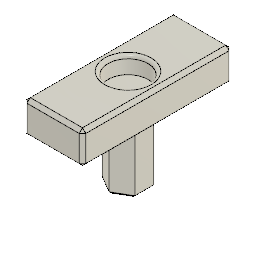
Hex Tool w magnet (Autodesk Fusion 360 design; units mm, degrees)
Autodesk Fusion 360 part; units mm, degrees
sketch "Sketch1" plane through (0, 0, 0) normal (0, 0, 1) x (1, 0, 0)
  line L0 (-2.5, -1.4434) -> (0, -2.8868)
  line L1 (0, -2.8868) -> (2.5, -1.4434)
  line L2 (2.5, -1.4434) -> (2.5, 1.4434)
  line L3 (2.5, 1.4434) -> (0, 2.8868)
  line L4 (0, 2.8868) -> (-2.5, 1.4434)
  line L5 (-2.5, 1.4434) -> (-2.5, -1.4434)
  dimension "d1" = 2.5
  constraint vertical L2
  measures "d1" distance of origin L5
extrude "Extrude1" add sketch "Sketch1" along normal blind 10 makes body 1
sketch "Sketch2" plane through (0, 0, 10) normal (0, 0, 1) x (-1, 0, 0)
  line L0 (2.5, -1.4434) -> (2.5, 1.4434)
  line L1 (2.5, 1.4434) -> (0, 2.8868)
  line L2 (0, 2.8868) -> (-2.5, 1.4434)
  line L3 (-2.5, 1.4434) -> (-2.5, -1.4434)
  line L4 (-2.5, -1.4434) -> (0, -2.8868)
  line L5 (0, -2.8868) -> (2.5, -1.4434)
  line L6 (2.5, -1.4434) -> (2.5, -11.4434)
  line L7 (2.5, -11.4434) -> (-2.5, -11.4434)
  line L8 (-2.5, -11.4434) -> (-2.5, -1.4434)
  line L9 (-2.5, 1.4434) -> (-2.5, 11.4434)
  line L10 (-2.5, 11.4434) -> (2.5, 11.4434)
  line L11 (2.5, 11.4434) -> (2.5, 1.4434)
  dimension "d4" = 5
  dimension "d5" = 5
  dimension "d6" = 10
  dimension "d7" = 10
  constraint coincident L0.start L5.end
  constraint vertical L6
  constraint perpendicular L6 L7
  constraint coincident L3.end L4.start
  constraint coincident L2.end L3.start
  constraint parallel L3 L9
  constraint perpendicular L9 L10
  constraint coincident L0.end L1.start
  measures "d4" distance of L9.end L10.end
  measures "d5" distance of L6.end L7.end
  measures "d6" distance of L10.end L0.end
  measures "d7" distance of L0.start L6.end
extrude "Extrude2" add sketch "Sketch2" along normal blind 5 separate body makes body 2
move_face "OffsetFaces1" offset 2 6 faces at (2.5, -0.4811, 11.6667) (2.5, 8.11, 11.6667) (2.5, -4.7767, 11.6667) (-2.5, 4.7767, 11.6667) (-2.5, 0.4811, 11.6667) (-2.5, -8.11, 11.6667) on bodies 2
combine "Combine1" operation add target body 1 tool bodies 2
sketch "Sketch3" plane through (0, 0, 15) normal (0, 0, 1) x (-1, 0, 0)
  line L0 (-4.5, 11.4434) -> (-4.5, -11.4434)
  line L1 (-4.5, -11.4434) -> (4.5, -11.4434)
  line L2 (4.5, -11.4434) -> (4.5, 11.4434)
  line L3 (4.5, 11.4434) -> (-4.5, 11.4434)
  circle A0 centre (0, 0) radius 3.05
  dimension "d11" = 6.1
  constraint coincident A0.centre origin
  measures "d11" diameter of A0
extrude "Extrude3" cut sketch "Sketch3" against normal blind 2.6 contours A0 bodies 1
fillet "Fillet1" radius 0.5 1 edges at (2.8436, -1.1029, 15) on bodies 1
chamfer "Chamfer1" distance 0.5 angle 45 12 edges at (0, -11.4434, 15) (4.5, 0, 15) (0, 11.4434, 15) (-4.5, 0, 15) (-4.5, 0, 10) (0, 11.4434, 10) (4.5, 0, 10) (4.5, -11.4434, 12.5) (0, -11.4434, 10) (4.5, 11.4434, 12.5) (-4.5, 11.4434, 12.5) (-4.5, -11.4434, 12.5) on bodies 1
chamfer "Chamfer2" distance 1 angle 45 6 edges at (1.25, -2.1651, 10) (2.5, 0, 10) (1.25, 2.1651, 10) (-1.25, 2.1651, 10) (-2.5, 0, 10) (-1.25, -2.1651, 10) on bodies 1
sketch "Sketch4" plane through (-4.5, 0, 0) normal (-1, 0, 0) x (0, -1, 0)
  line L0 (-10.9434, 10.5) -> (10.9434, 10.5)
  line L1 (10.9434, 10.5) -> (10.9434, 14.5)
  line L2 (10.9434, 14.5) -> (-10.9434, 14.5)
  line L3 (-10.9434, 14.5) -> (-10.9434, 10.5)
  spline S0 degree 2 poles (6.6137, 13.7758) (6.8028, 13.7758) (6.9498, 13.7019) knots 0 0 0 1 1 1
  spline S1 degree 2 poles (6.9498, 13.7019) (7.0968, 13.6279) (7.1888, 13.4869) knots 0 0 0 1 1 1
  spline S2 degree 2 poles (7.1888, 13.4869) (7.2808, 13.3459) (7.3117, 13.1482) knots 0 0 0 1 1 1
  line L4 (7.3117, 13.1482) -> (7.3117, 13.1465)
  line L5 (7.3117, 13.1465) -> (6.961, 13.1465)
  line L6 (6.961, 13.1465) -> (6.961, 13.1482)
  spline S3 degree 2 poles (6.961, 13.1482) (6.9421, 13.2858) (6.8509, 13.3623) knots 0 0 0 1 1 1
  spline S4 degree 2 poles (6.8509, 13.3623) (6.7598, 13.4388) (6.6137, 13.4388) knots 0 0 0 1 1 1
  spline S5 degree 2 poles (6.6137, 13.4388) (6.4452, 13.4388) (6.3532, 13.3262) knots 0 0 0 1 1 1
  spline S6 degree 2 poles (6.3532, 13.3262) (6.2612, 13.2135) (6.2612, 13.0089) knots 0 0 0 1 1 1
  line L7 (6.2612, 13.0089) -> (6.2612, 12.7992)
  spline S7 degree 2 poles (6.2612, 12.7992) (6.2612, 12.5963) (6.3532, 12.4837) knots 0 0 0 1 1 1
  spline S8 degree 2 poles (6.3532, 12.4837) (6.4452, 12.371) (6.6137, 12.371) knots 0 0 0 1 1 1
  spline S9 degree 2 poles (6.6137, 12.371) (6.7048, 12.371) (6.789, 12.4226) knots 0 0 0 1 1 1
  spline S10 degree 2 poles (6.789, 12.4226) (6.8733, 12.4742) (6.9369, 12.5671) knots 0 0 0 1 1 1
  line L8 (6.9369, 12.5671) -> (7.2567, 12.5671)
  line L9 (7.2567, 12.5671) -> (7.2567, 11.25)
  line L10 (7.2567, 11.25) -> (5.9826, 11.25)
  line L11 (5.9826, 11.25) -> (5.9826, 11.5836)
  line L12 (5.9826, 11.5836) -> (6.9059, 11.5836)
  line L13 (6.9059, 11.5836) -> (6.9059, 12.1458)
  spline S11 degree 2 poles (6.9059, 12.1458) (6.8406, 12.0925) (6.7598, 12.0633) knots 0 0 0 1 1 1
  spline S12 degree 2 poles (6.7598, 12.0633) (6.679, 12.034) (6.5947, 12.034) knots 0 0 0 1 1 1
  spline S13 degree 2 poles (6.5947, 12.034) (6.3781, 12.034) (6.2242, 12.1235) knots 0 0 0 1 1 1
  spline S14 degree 2 poles (6.2242, 12.1235) (6.0703, 12.2129) (5.9904, 12.3848) knots 0 0 0 1 1 1
  spline S15 degree 2 poles (5.9904, 12.3848) (5.9104, 12.5567) (5.9104, 12.7992) knots 0 0 0 1 1 1
  line L14 (5.9104, 12.7992) -> (5.9104, 13.0089)
  spline S16 degree 2 poles (5.9104, 13.0089) (5.9104, 13.2514) (5.9929, 13.4233) knots 0 0 0 1 1 1
  spline S17 degree 2 poles (5.9929, 13.4233) (6.0755, 13.5953) (6.2337, 13.6855) knots 0 0 0 1 1 1
  spline S18 degree 2 poles (6.2337, 13.6855) (6.3918, 13.7758) (6.6137, 13.7758) knots 0 0 0 1 1 1
  spline S19 degree 2 poles (3.2454, 12.6685) (3.2454, 12.4794) (3.3434, 12.3762) knots 0 0 0 1 1 1
  spline S20 degree 2 poles (3.3434, 12.3762) (3.4414, 12.273) (3.6185, 12.273) knots 0 0 0 1 1 1
  spline S21 degree 2 poles (3.6185, 12.273) (3.7818, 12.273) (3.8712, 12.3728) knots 0 0 0 1 1 1
  spline S22 degree 2 poles (3.8712, 12.3728) (3.9606, 12.4725) (3.9606, 12.6547) knots 0 0 0 1 1 1
  line L15 (3.9606, 12.6547) -> (4.0311, 12.3109)
  spline S23 degree 2 poles (4.0311, 12.3109) (3.9469, 12.1338) (3.8085, 12.0366) knots 0 0 0 1 1 1
  spline S24 degree 2 poles (3.8085, 12.0366) (3.67, 11.9395) (3.5033, 11.9395) knots 0 0 0 1 1 1
  spline S25 degree 2 poles (3.5033, 11.9395) (3.3107, 11.9395) (3.174, 12.0246) knots 0 0 0 1 1 1
  spline S26 degree 2 poles (3.174, 12.0246) (3.0373, 12.1097) (2.966, 12.273) knots 0 0 0 1 1 1
  spline S27 degree 2 poles (2.966, 12.273) (2.8946, 12.4364) (2.8946, 12.6668) knots 0 0 0 1 1 1
  line L16 (2.8946, 12.6668) -> (2.8946, 13.75)
  line L17 (2.8946, 13.75) -> (3.2454, 13.75)
  line L18 (3.2454, 13.75) -> (3.2454, 12.6685)
  line L19 (5.3774, 11.9653) -> (5.0267, 11.9653)
  line L20 (5.0267, 11.9653) -> (5.0267, 13.75)
  line L21 (5.0267, 13.75) -> (5.3774, 13.75)
  line L22 (5.3774, 13.75) -> (5.3774, 11.9653)
  spline S28 degree 2 poles (4.3114, 12.6685) (4.3114, 12.4794) (4.4042, 12.3762) knots 0 0 0 1 1 1
  spline S29 degree 2 poles (4.4042, 12.3762) (4.4971, 12.273) (4.6673, 12.273) knots 0 0 0 1 1 1
  spline S30 degree 2 poles (4.6673, 12.273) (4.8392, 12.273) (4.9329, 12.3642) knots 0 0 0 1 1 1
  spline S31 degree 2 poles (4.9329, 12.3642) (5.0267, 12.4553) (5.0267, 12.6204) knots 0 0 0 1 1 1
  line L23 (5.0267, 12.6204) -> (5.0628, 12.2765)
  spline S32 degree 2 poles (5.0628, 12.2765) (4.9802, 12.1149) (4.847, 12.0272) knots 0 0 0 1 1 1
  spline S33 degree 2 poles (4.847, 12.0272) (4.7137, 11.9395) (4.5521, 11.9395) knots 0 0 0 1 1 1
  spline S34 degree 2 poles (4.5521, 11.9395) (4.3647, 11.9395) (4.2323, 12.0246) knots 0 0 0 1 1 1
  spline S35 degree 2 poles (4.2323, 12.0246) (4.0999, 12.1097) (4.0303, 12.273) knots 0 0 0 1 1 1
  spline S36 degree 2 poles (4.0303, 12.273) (3.9606, 12.4364) (3.9606, 12.6668) knots 0 0 0 1 1 1
  line L24 (3.9606, 12.6668) -> (3.9606, 13.75)
  line L25 (3.9606, 13.75) -> (4.3114, 13.75)
  line L26 (4.3114, 13.75) -> (4.3114, 12.6685)
  spline S37 degree 2 poles (0.2295, 12.6685) (0.2295, 12.4794) (0.3275, 12.3762) knots 0 0 0 1 1 1
  spline S38 degree 2 poles (0.3275, 12.3762) (0.4255, 12.273) (0.6026, 12.273) knots 0 0 0 1 1 1
  spline S39 degree 2 poles (0.6026, 12.273) (0.766, 12.273) (0.8554, 12.3728) knots 0 0 0 1 1 1
  spline S40 degree 2 poles (0.8554, 12.3728) (0.9448, 12.4725) (0.9448, 12.6547) knots 0 0 0 1 1 1
  line L27 (0.9448, 12.6547) -> (1.0153, 12.3109)
  spline S41 degree 2 poles (1.0153, 12.3109) (0.9311, 12.1338) (0.7926, 12.0366) knots 0 0 0 1 1 1
  spline S42 degree 2 poles (0.7926, 12.0366) (0.6542, 11.9395) (0.4874, 11.9395) knots 0 0 0 1 1 1
  spline S43 degree 2 poles (0.4874, 11.9395) (0.2949, 11.9395) (0.1582, 12.0246) knots 0 0 0 1 1 1
  spline S44 degree 2 poles (0.1582, 12.0246) (0.0215, 12.1097) (-0.0499, 12.273) knots 0 0 0 1 1 1
  spline S45 degree 2 poles (-0.0499, 12.273) (-0.1212, 12.4364) (-0.1212, 12.6668) knots 0 0 0 1 1 1
  line L28 (-0.1212, 12.6668) -> (-0.1212, 13.75)
  line L29 (-0.1212, 13.75) -> (0.2295, 13.75)
  line L30 (0.2295, 13.75) -> (0.2295, 12.6685)
  line L31 (2.3616, 11.9653) -> (2.0108, 11.9653)
  line L32 (2.0108, 11.9653) -> (2.0108, 13.75)
  line L33 (2.0108, 13.75) -> (2.3616, 13.75)
  line L34 (2.3616, 13.75) -> (2.3616, 11.9653)
  spline S46 degree 2 poles (1.2956, 12.6685) (1.2956, 12.4794) (1.3884, 12.3762) knots 0 0 0 1 1 1
  spline S47 degree 2 poles (1.3884, 12.3762) (1.4813, 12.273) (1.6515, 12.273) knots 0 0 0 1 1 1
  spline S48 degree 2 poles (1.6515, 12.273) (1.8234, 12.273) (1.9171, 12.3642) knots 0 0 0 1 1 1
  spline S49 degree 2 poles (1.9171, 12.3642) (2.0108, 12.4553) (2.0108, 12.6204) knots 0 0 0 1 1 1
  line L35 (2.0108, 12.6204) -> (2.0469, 12.2765)
  spline S50 degree 2 poles (2.0469, 12.2765) (1.9644, 12.1149) (1.8312, 12.0272) knots 0 0 0 1 1 1
  spline S51 degree 2 poles (1.8312, 12.0272) (1.6979, 11.9395) (1.5363, 11.9395) knots 0 0 0 1 1 1
  spline S52 degree 2 poles (1.5363, 11.9395) (1.3489, 11.9395) (1.2165, 12.0246) knots 0 0 0 1 1 1
  spline S53 degree 2 poles (1.2165, 12.0246) (1.0841, 12.1097) (1.0144, 12.273) knots 0 0 0 1 1 1
  spline S54 degree 2 poles (1.0144, 12.273) (0.9448, 12.4364) (0.9448, 12.6668) knots 0 0 0 1 1 1
  line L36 (0.9448, 12.6668) -> (0.9448, 13.75)
  line L37 (0.9448, 13.75) -> (1.2956, 13.75)
  line L38 (1.2956, 13.75) -> (1.2956, 12.6685)
  line L39 (-3.0545, 11.25) -> (-3.4053, 11.25)
  line L40 (-3.4053, 11.25) -> (-3.4053, 13.75)
  line L41 (-3.4053, 13.75) -> (-3.0545, 13.75)
  line L42 (-3.0545, 13.75) -> (-3.0545, 11.25)
  line L43 (-1.6343, 11.25) -> (-1.985, 11.25)
  line L44 (-1.985, 11.25) -> (-1.985, 13.75)
  line L45 (-1.985, 13.75) -> (-1.6343, 13.75)
  line L46 (-1.6343, 13.75) -> (-1.6343, 11.25)
  line L47 (-1.8526, 12.3521) -> (-3.2402, 12.3521)
  line L48 (-3.2402, 12.3521) -> (-3.2402, 12.6857)
  line L49 (-3.2402, 12.6857) -> (-1.8526, 12.6857)
  line L50 (-1.8526, 12.6857) -> (-1.8526, 12.3521)
  spline S55 degree 2 poles (-4.7206, 13.7758) (-4.473, 13.7758) (-4.2976, 13.6829) knots 0 0 0 1 1 1
  spline S56 degree 2 poles (-4.2976, 13.6829) (-4.1222, 13.5901) (-4.0303, 13.4104) knots 0 0 0 1 1 1
  spline S57 degree 2 poles (-4.0303, 13.4104) (-3.9383, 13.2307) (-3.9383, 12.9763) knots 0 0 0 1 1 1
  line L51 (-3.9383, 12.9763) -> (-3.9383, 12.7751)
  spline S58 degree 2 poles (-3.9383, 12.7751) (-3.9383, 12.5103) (-4.0268, 12.3229) knots 0 0 0 1 1 1
  spline S59 degree 2 poles (-4.0268, 12.3229) (-4.1154, 12.1355) (-4.2839, 12.0375) knots 0 0 0 1 1 1
  spline S60 degree 2 poles (-4.2839, 12.0375) (-4.4524, 11.9395) (-4.6896, 11.9395) knots 0 0 0 1 1 1
  spline S61 degree 2 poles (-4.6896, 11.9395) (-4.9132, 11.9395) (-5.0714, 12.0512) knots 0 0 0 1 1 1
  spline S62 degree 2 poles (-5.0714, 12.0512) (-5.2295, 12.163) (-5.3129, 12.3745) knots 0 0 0 1 1 1
  spline S63 degree 2 poles (-5.3129, 12.3745) (-5.3963, 12.586) (-5.3963, 12.8817) knots 0 0 0 1 1 1
  line L52 (-5.3963, 12.8817) -> (-5.3963, 12.9986)
  line L53 (-5.3963, 12.9986) -> (-4.1927, 12.9986)
  line L54 (-4.1927, 12.9986) -> (-4.1927, 12.7166)
  line L55 (-4.1927, 12.7166) -> (-5.0628, 12.7166)
  spline S64 degree 2 poles (-5.0628, 12.7166) (-5.0473, 12.4983) (-4.9501, 12.3771) knots 0 0 0 1 1 1
  spline S65 degree 2 poles (-4.9501, 12.3771) (-4.853, 12.2558) (-4.6896, 12.2558) knots 0 0 0 1 1 1
  spline S66 degree 2 poles (-4.6896, 12.2558) (-4.4902, 12.2558) (-4.381, 12.3865) knots 0 0 0 1 1 1
  spline S67 degree 2 poles (-4.381, 12.3865) (-4.2718, 12.5172) (-4.2718, 12.7562) knots 0 0 0 1 1 1
  line L56 (-4.2718, 12.7562) -> (-4.2718, 12.9832)
  spline S68 degree 2 poles (-4.2718, 12.9832) (-4.2718, 13.205) (-4.3888, 13.3236) knots 0 0 0 1 1 1
  spline S69 degree 2 poles (-4.3888, 13.3236) (-4.5057, 13.4422) (-4.7206, 13.4422) knots 0 0 0 1 1 1
  spline S70 degree 2 poles (-4.7206, 13.4422) (-4.8272, 13.4422) (-4.9321, 13.3992) knots 0 0 0 1 1 1
  spline S71 degree 2 poles (-4.9321, 13.3992) (-5.037, 13.3563) (-5.1195, 13.2789) knots 0 0 0 1 1 1
  line L57 (-5.1195, 13.2789) -> (-5.3499, 13.5093)
  spline S72 degree 2 poles (-5.3499, 13.5093) (-5.2175, 13.6365) (-5.0524, 13.7062) knots 0 0 0 1 1 1
  spline S73 degree 2 poles (-5.0524, 13.7062) (-4.8874, 13.7758) (-4.7206, 13.7758) knots 0 0 0 1 1 1
  line L58 (-6.3901, 12.9384) -> (-5.7333, 11.9653)
  line L59 (-5.7333, 11.9653) -> (-6.1236, 11.9653)
  line L60 (-6.1236, 11.9653) -> (-6.636, 12.7648)
  line L61 (-6.636, 12.7648) -> (-7.3117, 13.75)
  line L62 (-7.3117, 13.75) -> (-6.9231, 13.75)
  line L63 (-6.9231, 13.75) -> (-6.3901, 12.9384)
  line L64 (-6.3798, 12.7648) -> (-6.5483, 13.088)
  line L65 (-6.5483, 13.088) -> (-6.0944, 13.75)
  line L66 (-6.0944, 13.75) -> (-5.7058, 13.75)
  line L67 (-5.7058, 13.75) -> (-6.3798, 12.7648)
  line L68 (-6.5036, 12.598) -> (-6.8939, 11.9653)
  line L69 (-6.8939, 11.9653) -> (-7.2842, 11.9653)
  line L70 (-7.2842, 11.9653) -> (-6.6515, 12.9281)
  line L71 (-6.6515, 12.9281) -> (-6.5036, 12.598)
extrude "Extrude4" cut sketch "Sketch4" against normal blind 0.2 contours S0 S1 S2 L5 S3 S4 S5 S6 L7 S7 S8 S9 S10 L8 L9 L10 L11 L12 L13 S11 S12 S13 S14 S15 L14 S16 S17 S18 | S19 S20 S21 S22 S23 S24 S25 S26 S27 L16 L17 L18 S36 | L15 S23 L20 S28 S29 S30 S31 S32 S33 S34 S35 S36 L24 L25 L26 | L15 S23 S36 | L19 L20 L21 L22 L23 S32 | L20 L23 S32 | S37 S38 S39 S40 S41 S42 S43 S44 S45 L28 L29 L30 S54 | L27 S41 L32 S46 S47 S48 S49 S50 S51 S52 S53 S54 L36 L37 L38 | L27 S41 S54 | L31 L32 L33 L34 L35 S50 | L32 L35 S50 | L39 L40 L41 L42 L47 L48 L49 | L42 L47 L48 L49 | L42 L44 L47 L49 | L43 L44 L45 L46 L47 L49 L50 | L44 L47 L49 L50 | L53 L54 L55 S67 L56 S68 | S55 S56 S57 L51 S58 S59 S60 S61 S62 S63 L52 L53 S68 S69 S70 S71 L57 S72 S73 | L58 L63 L65 L66 L67 | L58 L63 L64 L65 L67 | L58 L59 L60 L61 L62 L63 L64 L65 L67 L68 L70 L71 | L60 L61 L68 L69 L70 | L60 L61 L68 L70 L71 bodies 1
chamfer "Chamfer3" distance 0.5 angle 45 6 edges at (-1.25, 2.1651, 0) (1.25, 2.1651, 0) (2.5, 0, 0) (1.25, -2.1651, 0) (-1.25, -2.1651, 0) (-2.5, 0, 0) on bodies 1
